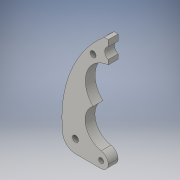
# Autodesk Inventor part: left finger JR
Saved by Autodesk Inventor 2016 (Build 200138000, 138)
## iProperties
Created: 2016-05-23
Part Number: left finger JR
Material: Generic
Document SubType Name: Modeling
Designer: jregalado
Density: 1 g/cm^3
Appearance: Default
Author: jregalado
Autodesk Inventor part; units mm, degrees
ref_plane "YZ Plane" through (0, 0, 0) normal (1, 0, 0) x (0, 1, 0)
ref_plane "XZ Plane" through (0, 0, 0) normal (0, 1, 0) x (-1, 0, 0)
ref_plane "XY Plane" through (0, 0, 0) normal (0, 0, 1) x (1, 0, 0)
sketch "Sketch1" plane through (0, 0, 0) normal (0, 0, 1) x (1, 0, 0)
  arc A0 (-43.0429, 56.0067) -> (-69.1121, -14.5933) centre (0, 0) ccw
  arc A1 (-52.0889, 15.1517) -> (-43.0429, -5.2586) centre (-45.4399, 5.8888) ccw
  line L0 (-69.1121, -14.5933) -> (-43.0429, -14.5933)
  line L1 (-43.0429, 56.0067) -> (-43.0429, 41.0384)
  line L2 (-43.0429, -5.2586) -> (-43.0429, -14.5933)
  arc A2 (-43.0429, 41.0384) -> (-52.0889, 15.1517) centre (-41.6223, 26.0181) ccw
  line L3 (-43.0429, -0.3022) -> (-43.0429, -3.0397)
  dimension "d0" = 141.272
  dimension "d5" = 22.8043
  dimension "d6" = 5.8888
  dimension "d7" = 26.0181
  dimension "d8" = 14.5933
  dimension "d33" = 15.0873
  dimension "d35" = 2.7376
  dimension "d36" = 0.3022
  constraints: 8 end point, 6 point on circle, 3 centre point, 2 point on line, 2 vertical, 1 coincident, 1 horizontal
  measures "d0" diameter of A0
  measures "d5" diameter of A1
  measures "d6" vertical distance of A1.centre point (0, 0)
  measures "d7" vertical distance of point (0, 0) A2.centre
  measures "d8" distance from line of L0 point (0, 0)
  measures "d33" radius of A2
  measures "d35" distance of L3.start L3.end
  measures "d36" vertical distance of point (0, 0) L3.start
extrude "Extrusion1" add sketch "Sketch1" along normal blind 5.83
fillet "Fillet1" radius 7.8 1 edges at (-69.1121, -14.5933, 2.915)
fillet "Fillet2" radius 4.33 1 edges at (-43.0429, -14.5933, 2.915)
sketch "Sketch2" plane through (0, 0, 5.83) normal (0, 0, 1) x (1, 0, 0)
  circle A0 centre (-41.6223, 47.1026) radius 3.565
  line L0 (-43.0429, 41.0384) -> (-43.0429, 56.0067) projected
  point P0 (0, 0)
  point P1 (-43.0429, -10.2633)
  dimension "d14" = 1.4206
  dimension "d15" = 7.13
  dimension "d32" = 47.1026
  constraints: 1 centre point
  measures "d14" distance from line of L0 A0.centre
  measures "d15" diameter of A0
  measures "d32" vertical distance of point (0, 0) A0.centre
extrude "Extrusion2" cut sketch "Sketch2" against normal through all
sketch "Sketch3" plane through (0, 0, 5.83) normal (0, 0, 1) x (1, 0, 0)
  arc A0 (-43.0429, 56.0067) -> (-70.222, -7.6365) centre (0, 0) ccw projected
  line L0 (-45.4131, 54.1026) -> (-43.0429, 54.1026)
  line L1 (-43.0429, 50.3723) -> (-43.0429, 56.0067) projected
  line L2 (-43.0429, 56.0067) -> (-43.0429, 54.1026)
  arc A1 (-43.0429, 56.0067) -> (-45.4131, 54.1026) centre (0, 0) ccw
  dimension "d18" = 54.1026
  constraints: 4 end point, 3 point on circle, 1 centre point, 1 coincident, 1 concentric, 1 horizontal, 1 perpendicular
  measures "d18" distance from line of point (0, 0) L0
extrude "Extrusion3" cut sketch "Sketch3" against normal through all
sketch "Sketch4" plane through (0, 0, 5.83) normal (0, 0, 1) x (1, 0, 0)
  circle A0 centre (-52.0304, 42.0841) radius 1.725
  circle A1 centre (-62.564, -6.7927) radius 1.8
  circle A2 centre (-47.2872, -10.4133) radius 1.5
  point P0 (0, 0)
  dimension "d21" = 10.4133
  dimension "d22" = 6.7927
  dimension "d23" = 42.0841
  dimension "d24" = 47.2872
  dimension "d25" = 62.564
  dimension "d26" = 52.0304
  dimension "d27" = 3
  dimension "d28" = 3.6
  dimension "d29" = 3.45
  constraints: 3 centre point
  measures "d21" vertical distance of point (0, 0) A2.centre
  measures "d22" vertical distance of point (0, 0) A1.centre
  measures "d23" vertical distance of point (0, 0) A0.centre
  measures "d24" horizontal distance of point (0, 0) A2.centre
  measures "d25" horizontal distance of point (0, 0) A1.centre
  measures "d26" horizontal distance of point (0, 0) A0.centre
  measures "d27" diameter of A2
  measures "d28" diameter of A1
  measures "d29" diameter of A0
extrude "Extrusion4" cut sketch "Sketch4" against normal through all
fillet "Fillet4" radius 5.0505 1 edges at (-43.0429, -5.2586, 2.915)
body "Solid1"
